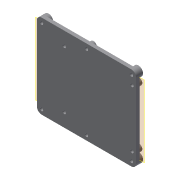
# Autodesk Inventor part: cellSTORM_v5_Electronicbox
Saved by Autodesk Inventor 2019 (Build 230136000, 136)
## iProperties
Created: 2020-05-04
Part Number: cellSTORM_v5_Electronicbox
Material: Generic
Document SubType Name: Modeling
Designer: diederichbenedict
Density: 1 g/cm^3
Appearance: Default
Author: diederichbenedict
Autodesk Inventor part; units mm, degrees
ref_plane "YZ Plane" through (0, 0, 0) normal (1, 0, 0) x (0, 1, 0)
ref_plane "XZ Plane" through (0, 0, 0) normal (0, 1, 0) x (-1, 0, 0)
ref_plane "XY Plane" through (0, 0, 0) normal (0, 0, 1) x (1, 0, 0)
ref_plane "Work Plane1" through (0, 0, 3.25) normal (0, 0, 1) x (1, 0, 0)
sketch "Sketch1" plane through (0, 0, 3.25) normal (0, 0, 1) x (1, 0, 0)
  arc A0 (3, 0) -> (0, -3) centre (3, -3) ccw construction
  arc A1 (81.9242, -56) -> (84.9242, -53) centre (81.9242, -53) ccw construction
  arc A2 (84.9242, -3) -> (81.9242, 0) centre (81.9242, -3) ccw construction
  arc A3 (0, -53) -> (3, -56) centre (3, -53) ccw construction
  line L0 (0, 0) -> (86.0371, 0) construction
  line L1 (86.0371, 0) -> (86.0371, -52.7339) construction
  line L2 (86.0371, -52.7339) -> (0, -52.7339) construction
  line L3 (0, -52.7339) -> (0, 0) construction
  line L4 (80.9242, -64) -> (4, -64)
  line L5 (0, -60) -> (0, 4)
  line L6 (4, 8) -> (80.9242, 8)
  line L7 (84.9242, 4) -> (84.9242, -60)
  circle A4 centre (23.4242, -3.5) radius 1.375 projected
  circle A5 centre (23.4242, -52.5) radius 1.375 projected
  circle A6 centre (81.4242, -52.5) radius 1.375 projected
  circle A7 centre (81.4242, -3.5) radius 1.375 projected
  arc A8 (4, 8) -> (0, 4) centre (4, 4) ccw
  arc A9 (0, -60) -> (4, -64) centre (4, -60) ccw
  arc A10 (80.9242, -64) -> (84.9242, -60) centre (80.9242, -60) ccw
  arc A11 (84.9242, 4) -> (80.9242, 8) centre (80.9242, 4) ccw
  circle A12 centre (42.4621, 4) radius 1.4
  circle A13 centre (4, 4) radius 1.4
  circle A14 centre (4, -60) radius 1.4
  circle A15 centre (42.4621, -60) radius 1.4
  circle A16 centre (80.9242, -60) radius 1.4
  circle A17 centre (80.9242, 4) radius 1.4
  point P0 (84.9242, -64)
  point P1 (0, 8)
  point P2 (0, -64)
  point P3 (84.9242, 8)
  dimension "d0" = 8
  dimension "d2" = 0
  dimension "d5" = 4
  dimension "d12" = 8
  dimension "d13" = 2.8
  dimension "d14" = 2.8
  dimension "d15" = 2.8
  dimension "d16" = 2.8
  dimension "d17" = 2.8
  dimension "d18" = 2.8
  constraints: 16 end point, 10 centre point, 8 point on circle, 8 point on line, 8 tangent, 6 coincident, 4 parallel, 3 equal radius, 2 horizontal, 2 perpendicular
  measures "d0" distance between parallel lines of L6 L0
  measures "d2" distance from line of A1.end L7
  measures "d5" radius of A8
  measures "d12" vertical distance of A3.end L4.end
  measures "d13" diameter of A12
  measures "d14" diameter of A13
  measures "d15" diameter of A14
  measures "d16" diameter of A15
  measures "d17" diameter of A16
  measures "d18" diameter of A17
extrude "Extrusion1" add sketch "Sketch1" along normal blind 3
sketch "Sketch2" plane through (0, 0, 3.25) normal (0, 0, -1) x (-1, 0, 0)
  circle A0 centre (-23.4242, -3.5) radius 1.375 projected
  circle A1 centre (-23.4242, -52.5) radius 1.375 projected
  arc A2 (-3, -56) -> (0, -53) centre (-3, -53) ccw projected
  line L0 (0, -3) -> (0, -53) projected
  arc A3 (0, -3) -> (-3, 0) centre (-3, -3) ccw projected
  line L1 (-81.9242, 0) -> (-3, 0) projected
  arc A4 (-81.9242, 0) -> (-84.9242, -3) centre (-81.9242, -3) ccw projected
  line L2 (-84.9242, -53) -> (-84.9242, -3) projected
  arc A5 (-84.9242, -53) -> (-81.9242, -56) centre (-81.9242, -53) ccw projected
  line L3 (-3, -56) -> (-81.9242, -56) projected
  circle A6 centre (-22.213, -8.2226) radius 0.5 projected
  circle A7 centre (-24.7543, -8.2226) radius 0.5 projected
  circle A8 centre (-67.0848, -6.0884) radius 0.2 projected
  circle A9 centre (-48.353, -16.7207) radius 0.2 projected
  circle A10 centre (-47.3865, -17.6798) radius 0.2 projected
  circle A11 centre (-45.8783, -17.6652) radius 0.2 projected
  circle A12 centre (-44.8533, -17.6652) radius 0.2 projected
  circle A13 centre (-46.2005, -16.2668) radius 0.2 projected
  circle A14 centre (-45.5781, -16.2009) radius 0.2 projected
  circle A15 centre (-44.9045, -16.1936) radius 0.2 projected
  circle A16 centre (-44.2822, -16.3107) radius 0.2 projected
  circle A17 centre (-43.9225, -35.8663) radius 0.2 projected
  circle A18 centre (-43.7816, -34.9329) radius 0.2 projected
  circle A19 centre (-44.7326, -34.6159) radius 0.2 projected
  circle A20 centre (-46.2119, -33.2071) radius 0.2 projected
  circle A21 centre (-43.4822, -31.4107) radius 0.2 projected
  circle A22 centre (-38.8402, -21.8362) radius 0.2 projected
  circle A23 centre (-38.8242, -20.7804) radius 0.2 projected
  circle A24 centre (-36.9127, -18.1491) radius 0.2 projected
  circle A25 centre (-37.5765, -17.9571) radius 0.2 projected
  circle A26 centre (-37.0167, -19.0928) radius 0.2 projected
  circle A27 centre (-38.1204, -19.9646) radius 0.2 projected
  line L4 (-38.4822, -15.9107) -> (-37.8289, -15.9107) projected
  line L5 (-37.8289, -16.3532) -> (-37.8289, -15.9107) projected
  line L6 (-37.8289, -16.3532) -> (-38.4822, -16.3532) projected
  line L7 (-38.4822, -15.9107) -> (-38.4822, -16.3532) projected
  line L8 (-38.5091, -16.758) -> (-37.8127, -16.758) projected
  line L9 (-37.8127, -17.341) -> (-37.8127, -16.758) projected
  line L10 (-37.8127, -17.341) -> (-38.5091, -17.341) projected
  line L11 (-38.5091, -16.758) -> (-38.5091, -17.341) projected
  circle A28 centre (-72.081, -8.9661) radius 0.2 projected
  circle A29 centre (-79.5495, -9.7485) radius 0.2 projected
  circle A30 centre (-79.9051, -8.7527) radius 0.2 projected
  circle A31 centre (-77.6646, -9.4996) radius 0.2 projected
  circle A32 centre (-79.7806, -11.3489) radius 0.2 projected
  circle A33 centre (-79.3894, -12.807) radius 0.2 projected
  circle A34 centre (-79.1761, -13.5361) radius 0.2 projected
  circle A35 centre (-70.8491, -11.3341) radius 0.2 projected
  circle A36 centre (-70.7681, -10.4839) radius 0.2 projected
  circle A37 centre (-71.8713, -11.4758) radius 0.2 projected
  circle A38 centre (-47.3628, -8.6438) radius 0.2 projected
  circle A39 centre (-67.9301, -8.3536) radius 0.2 projected
  circle A40 centre (-68.8541, -7.4295) radius 0.2 projected
  circle A41 centre (-64.6394, -6.3589) radius 0.2 projected
  circle A42 centre (-65.124, -8.6691) radius 0.2 projected
  circle A43 centre (-67.1863, -9.0861) radius 0.2 projected
  circle A44 centre (-66.6003, -9.8073) radius 0.2 projected
  circle A45 centre (-66.7693, -10.5962) radius 0.2 projected
  circle A46 centre (-66.8031, -11.2611) radius 0.2 projected
  circle A47 centre (-65.586, -10.9681) radius 0.2 projected
  circle A48 centre (-62.3629, -10.461) radius 0.2 projected
  circle A49 centre (-62.4756, -12.7825) radius 0.2 projected
  circle A50 centre (-64.7183, -13.8643) radius 0.2 projected
  circle A51 centre (-63.873, -13.8643) radius 0.2 projected
  circle A52 centre (-61.9347, -16.2197) radius 0.2 projected
  circle A53 centre (-59.9625, -15.3068) radius 0.2 projected
  circle A54 centre (-60.7965, -14.1573) radius 0.2 projected
  circle A55 centre (-58.7116, -11.0019) radius 0.2 projected
  circle A56 centre (-56.2098, -8.2183) radius 0.2 projected
  circle A57 centre (-55.1542, -11.3073) radius 0.2 projected
  circle A58 centre (-58.4406, -13.9483) radius 0.2 projected
  circle A59 centre (-57.6689, -13.9483) radius 0.2 projected
  circle A60 centre (-56.7841, -14.2211) radius 0.2 projected
  circle A61 centre (-56.345, -11.3738) radius 0.2 projected
  circle A62 centre (-43.0801, -22.1797) radius 0.2 projected
  circle A63 centre (-45.846, -22.8336) radius 0.2 projected
  circle A64 centre (-45.6957, -23.6153) radius 0.2 projected
  circle A65 centre (-47.4169, -23.2545) radius 0.2 projected
  circle A66 centre (-47.3794, -24.8404) radius 0.2 projected
  circle A67 centre (-47.7852, -23.7957) radius 0.2 projected
  circle A68 centre (-46.0339, -25.0509) radius 0.2 projected
  circle A69 centre (-37.8814, -28.3476) radius 0.2 projected
  circle A70 centre (-38.5166, -28.276) radius 0.2 projected
  circle A71 centre (-39.2056, -28.3208) radius 0.2 projected
  circle A72 centre (-38.123, -26.8266) radius 0.2 projected
  circle A73 centre (-38.9819, -26.8266) radius 0.2 projected
  circle A74 centre (-39.134, -25.3146) radius 0.2 projected
  circle A75 centre (-45.0926, -23.6057) radius 0.2 projected
  circle A76 centre (-39.805, -25.3146) radius 0.2 projected
  circle A77 centre (-40.306, -25.8693) radius 0.2 projected
  circle A78 centre (-73.2524, -44.2624) radius 0.2 projected
  circle A79 centre (-75.8766, -48.3708) radius 0.2 projected
  circle A80 centre (-74.335, -47.9589) radius 0.2 projected
  circle A81 centre (-75.6234, -44.5695) radius 0.2 projected
  circle A82 centre (-60.44, -36.6138) radius 0.2 projected
  circle A83 centre (-61.037, -35.3004) radius 0.2 projected
  circle A84 centre (-61.2076, -34.3622) radius 0.2 projected
  circle A85 centre (-64.6361, -37.0573) radius 0.2 projected
  circle A86 centre (-65.3014, -36.0338) radius 0.2 projected
  circle A87 centre (-64.6703, -33.3899) radius 0.2 projected
  circle A88 centre (-63.715, -39.9741) radius 0.2 projected
  circle A89 centre (-65.1479, -39.0018) radius 0.2 projected
  circle A90 centre (-68.8954, -35.575) radius 0.2 projected
  circle A91 centre (-69.402, -34.9183) radius 0.2 projected
  circle A92 centre (-69.8898, -36.0628) radius 0.2 projected
  circle A93 centre (-72.1039, -38.1643) radius 0.2 projected
  circle A94 centre (-71.935, -41.8794) radius 0.2 projected
  circle A95 centre (-72.1227, -34.7119) radius 0.2 projected
  circle A96 centre (-74.0553, -35.256) radius 0.2 projected
  circle A97 centre (-75.0685, -34.9558) radius 0.2 projected
  circle A98 centre (-77.5077, -35.1622) radius 0.2 projected
  circle A99 centre (-68.9517, -32.6104) radius 0.2 projected
  circle A100 centre (-66.6813, -30.8654) radius 0.2 projected
  circle A101 centre (-66.8877, -29.6458) radius 0.2 projected
  circle A102 centre (-44.52, -23.6415) radius 0.2 projected
  circle A103 centre (-45.0568, -24.8404) radius 0.2 projected
  circle A104 centre (-44.4842, -24.8225) radius 0.2 projected
  circle A105 centre (-43.8937, -24.8136) radius 0.2 projected
  circle A106 centre (-42.3638, -26.2988) radius 0.2 projected
  circle A107 centre (-43.7148, -26.2719) radius 0.2 projected
  circle A108 centre (-44.7079, -26.2719) radius 0.2 projected
  circle A109 centre (-44.1979, -26.7193) radius 0.2 projected
  circle A110 centre (-44.7705, -26.8445) radius 0.2 projected
  circle A111 centre (-41.5854, -28.2402) radius 0.2 projected
  circle A112 centre (-42.9543, -28.2134) radius 0.2 projected
  circle A113 centre (-44.2695, -28.3118) radius 0.2 projected
  circle A114 centre (-44.9763, -28.4192) radius 0.2 projected
  circle A115 centre (-45.3968, -26.6656) radius 0.2 projected
  circle A116 centre (-46.0142, -26.7551) radius 0.2 projected
  circle A117 centre (-47.6514, -26.3882) radius 0.2 projected
  circle A118 centre (-48.8593, -27.5961) radius 0.2 projected
  circle A119 centre (-55.7434, -31.6719) radius 0.2 projected
  circle A120 centre (-57.2346, -31.7216) radius 0.2 projected
  circle A121 centre (-56.4393, -32.9394) radius 0.2 projected
  circle A122 centre (-70.5072, -27.1836) radius 0.2 projected
  circle A123 centre (-82.0135, -8.0436) radius 0.2 projected
  circle A124 centre (-77.8638, -7.5634) radius 0.2 projected
  circle A125 centre (-77.3837, -6.7061) radius 0.2 projected
  circle A126 centre (-69.7875, -6.2774) radius 0.2 projected
  circle A127 centre (-70.8849, -6.6203) radius 0.2 projected
  circle A128 centre (-70.2762, -8.4294) radius 0.2 projected
  circle A129 centre (-72.6339, -6.5603) radius 0.2 projected
  circle A130 centre (-77.2174, -15.0208) radius 0.2 projected
  circle A131 centre (-74.5254, -13.0345) radius 0.2 projected
  circle A132 centre (-74.7215, -13.6095) radius 0.2 projected
  circle A133 centre (-74.2641, -14.1061) radius 0.2 projected
  circle A134 centre (-74.826, -14.6941) radius 0.2 projected
  circle A135 centre (-71.0103, -13.8709) radius 0.2 projected
  circle A136 centre (-70.9057, -14.6027) radius 0.2 projected
  circle A137 centre (-72.8789, -14.7856) radius 0.2 projected
  circle A138 centre (-72.2909, -15.1646) radius 0.2 projected
  circle A139 centre (-76.4202, -23.4755) radius 0.2 projected
  circle A140 centre (-76.6424, -22.9136) radius 0.2 projected
  circle A141 centre (-72.1341, -21.5546) radius 0.2 projected
  circle A142 centre (-71.337, -21.5938) radius 0.2 projected
  circle A143 centre (-75.414, -19.4507) radius 0.2 projected
  circle A144 centre (-77.335, -18.9933) radius 0.2 projected
  circle A145 centre (-73.0619, -16.7196) radius 0.2 projected
  circle A146 centre (-72.1733, -16.1838) radius 0.2 projected
  circle A147 centre (-70.7751, -16.1316) radius 0.2 projected
  circle A148 centre (-70.7881, -17.0724) radius 0.2 projected
  circle A149 centre (-71.7558, -44.5458) radius 0.2 projected
  circle A150 centre (-66.535, -44.9267) radius 0.2 projected
  circle A151 centre (-65.8404, -45.218) radius 0.2 projected
  circle A152 centre (-64.1151, -43.2014) radius 0.2 projected
  circle A153 centre (-67.1848, -42.3948) radius 0.2 projected
  circle A154 centre (-68.2379, -42.4172) radius 0.2 projected
  circle A155 centre (-80.9558, -44.2504) radius 0.2 projected
  circle A156 centre (-80.0692, -44.0164) radius 0.2 projected
  circle A157 centre (-83.899, -39.4107) radius 0.2 projected
  circle A158 centre (-83.9729, -38.6226) radius 0.2 projected
  circle A159 centre (-83.8374, -36.4183) radius 0.2 projected
  circle A160 centre (-78.5914, -39.5092) radius 0.2 projected
  circle A161 centre (-78.5791, -38.1177) radius 0.2 projected
  circle A162 centre (-77.8266, -25.7432) radius 0.2 projected
  circle A163 centre (-77.9087, -28.671) radius 0.2 projected
  circle A164 centre (-77.895, -31.7083) radius 0.2 projected
  circle A165 centre (-74.0916, -28.6573) radius 0.2 projected
  circle A166 centre (-77.6854, -23.1009) radius 0.2 projected
  circle A167 centre (-75.7973, -21.5412) radius 0.2 projected
  circle A168 centre (-70.7489, -18.0525) radius 0.2 projected
  circle A169 centre (-70.8584, -18.9144) radius 0.2 projected
  circle A170 centre (-70.7763, -19.5301) radius 0.2 projected
  circle A171 centre (-66.4667, -19.749) radius 0.2 projected
  circle A172 centre (-65.6666, -20.7133) radius 0.2 projected
  circle A173 centre (-71.5914, -22.7486) radius 0.2 projected
  circle A174 centre (-71.4444, -23.5627) radius 0.2 projected
  circle A175 centre (-72.2443, -23.8456) radius 0.2 projected
  circle A176 centre (-73.4429, -24.8971) radius 0.2 projected
  circle A177 centre (-68.4368, -27.26) radius 0.2 projected
  circle A178 centre (-73.2535, -29.6345) radius 0.2 projected
  circle A179 centre (-73.1065, -28.6847) radius 0.2 projected
  circle A180 centre (-71.125, -25.1459) radius 0.2 projected
  circle A181 centre (-71.1935, -25.8197) radius 0.2 projected
  circle A182 centre (-71.2849, -27.2245) radius 0.2 projected
  circle A183 centre (-71.1706, -29.5087) radius 0.2 projected
  circle A184 centre (-71.2278, -28.6864) radius 0.2 projected
  circle A185 centre (-66.8649, -27.1446) radius 0.2 projected
  circle A186 centre (-66.6593, -28.8235) radius 0.2 projected
  circle A187 centre (-66.5108, -30.2625) radius 0.2 projected
  circle A188 centre (-42.5801, -10.5439) radius 0.2 projected
  circle A189 centre (-41.6928, -10.461) radius 0.2 projected
  circle A190 centre (-40.7805, -10.4527) radius 0.2 projected
  circle A191 centre (-44.6203, -13.488) radius 0.2 projected
  circle A192 centre (-42.0825, -14.4002) radius 0.2 projected
  circle A193 centre (-45.491, -12.3933) radius 0.2 projected
  circle A194 centre (-44.5373, -12.4265) radius 0.2 projected
  circle A195 centre (-43.426, -12.4099) radius 0.2 projected
  circle A196 centre (-0.8218, -17.9959) radius 0.2 projected
  circle A197 centre (-5.3083, -17.8009) radius 0.2 projected
  circle A198 centre (-36.7643, -43.1201) radius 0.2 projected
  circle A199 centre (-19.8744, -38.9768) radius 0.2 projected
  circle A200 centre (-20.6732, -38.164) radius 0.2 projected
  circle A201 centre (-16.553, -31.5352) radius 0.2 projected
  circle A202 centre (-16.6371, -33.7074) radius 0.2 projected
  circle A203 centre (-17.4359, -35.4873) radius 0.2 projected
  circle A204 centre (-20.477, -31.0167) radius 0.2 projected
  circle A205 centre (-21.5701, -33.8896) radius 0.2 projected
  circle A206 centre (-31.4223, -28.9566) radius 0.2 projected
  circle A207 centre (-29.5724, -29.9936) radius 0.2 projected
  circle A208 centre (-28.8156, -27.3589) radius 0.2 projected
  circle A209 centre (-27.8906, -27.401) radius 0.2 projected
  circle A210 centre (-26.3911, -27.5551) radius 0.2 projected
  circle A211 centre (-24.8635, -27.485) radius 0.2 projected
  circle A212 centre (-24.1564, -30.0892) radius 0.2 projected
  circle A213 centre (-23.9144, -29.4776) radius 0.2 projected
  circle A214 centre (-22.8697, -30.1147) radius 0.2 projected
  circle A215 centre (-23.2009, -29.5541) radius 0.2 projected
  circle A216 centre (-23.1499, -27.4901) radius 0.2 projected
  circle A217 centre (-22.3218, -27.4901) radius 0.2 projected
  circle A218 centre (-21.2899, -27.401) radius 0.2 projected
  circle A219 centre (-20.5113, -27.5708) radius 0.2 projected
  circle A220 centre (-19.7893, -23.9044) radius 0.2 projected
  circle A221 centre (-19.761, -21.3705) radius 0.2 projected
  circle A222 centre (-19.4779, -20.7335) radius 0.2 projected
  circle A223 centre (-19.7893, -18.7941) radius 0.2 projected
  circle A224 centre (-19.945, -17.8598) radius 0.2 projected
  circle A225 centre (-21.2757, -16.7698) radius 0.2 projected
  circle A226 centre (-22.3799, -15.5949) radius 0.2 projected
  circle A227 centre (-24.7014, -15.6232) radius 0.2 projected
  circle A228 centre (-29.8825, -15.7648) radius 0.2 projected
  circle A229 centre (-35.6443, -10.4124) radius 0.2 projected
  circle A230 centre (-37.175, -12.1575) radius 0.2 projected
  circle A231 centre (-39.8268, -12.6255) radius 0.2 projected
  circle A232 centre (-37.331, -14.1464) radius 0.2 projected
  circle A233 centre (-37.0872, -14.8191) radius 0.2 projected
  circle A234 centre (-38.3839, -15.2773) radius 0.2 projected
  circle A235 centre (-38.9688, -15.9012) radius 0.2 projected
  circle A236 centre (-40.636, -16.2522) radius 0.2 projected
  circle A237 centre (-41.2794, -16.301) radius 0.2 projected
  circle A238 centre (-39.7721, -19.9788) radius 0.2 projected
  circle A239 centre (-41.478, -19.3199) radius 0.2 projected
  circle A240 centre (-42.2322, -19.9715) radius 0.2 projected
  circle A241 centre (-47.1376, -20.7183) radius 0.2 projected
  circle A242 centre (-44.8753, -21.326) radius 0.2 projected
  circle A243 centre (-45.7392, -20.8208) radius 0.2 projected
  circle A244 centre (-44.824, -20.7549) radius 0.2 projected
  circle A245 centre (-46.0467, -19.8031) radius 0.2 projected
  circle A246 centre (-45.439, -19.6201) radius 0.2 projected
  circle A247 centre (-44.4579, -19.686) radius 0.2 projected
  circle A248 centre (-44.7654, -19.1442) radius 0.2 projected
  circle A249 centre (-44.0479, -19.0417) radius 0.2 projected
  circle A250 centre (-42.364, -18.024) radius 0.2 projected
  circle A251 centre (-44.6117, -18.5511) radius 0.2 projected
  circle A252 centre (-47.3353, -19.254) radius 0.2 projected
  circle A253 centre (-42.3786, -18.844) radius 0.2 projected
  circle A254 centre (-45.8856, -18.4999) radius 0.2 projected
  circle A255 centre (-73.3884, -7.7263) radius 0.2 projected
  circle A256 centre (-73.2512, -8.8838) radius 0.2 projected
  circle A257 centre (-72.7822, -10.7673) radius 0.2 projected
  circle A258 centre (-72.747, -11.7788) radius 0.2 projected
  circle A259 centre (-73.7231, -11.767) radius 0.2 projected
  circle A260 centre (-76.5692, -10.5556) radius 0.2 projected
  circle A261 centre (-76.5339, -11.1437) radius 0.2 projected
  circle A262 centre (-76.7103, -12.1669) radius 0.2 projected
  circle A263 centre (-78.9449, -14.3897) radius 0.2 projected
  circle A264 centre (-72.9965, -18.0002) radius 0.2 projected
  circle A265 centre (-73.271, -19.5945) radius 0.2 projected
  circle A266 centre (-78.1452, -14.1192) radius 0.2 projected
  circle A267 centre (-77.4395, -14.1061) radius 0.2 projected
  circle A268 centre (-78.4065, -15.831) radius 0.2 projected
  circle A269 centre (-78.3673, -16.6412) radius 0.2 projected
  circle A270 centre (-77.8969, -17.4514) radius 0.2 projected
  circle A271 centre (-77.2304, -16.7065) radius 0.2 projected
  circle A272 centre (-76.2112, -15.5174) radius 0.2 projected
  circle A273 centre (-76.5901, -16.4321) radius 0.2 projected
  circle A274 centre (-77.0605, -15.7918) radius 0.2 projected
  circle A275 centre (-55.7793, -42.2185) radius 0.2 projected
  circle A276 centre (-57.5522, -41.3263) radius 0.2 projected
  circle A277 centre (-55.928, -40.3426) radius 0.2 projected
  circle A278 centre (-55.8365, -41.4178) radius 0.2 projected
  circle A279 centre (-55.8822, -43.1107) radius 0.2 projected
  circle A280 centre (-58.7419, -42.127) radius 0.2 projected
  circle A281 centre (-59.3824, -38.5924) radius 0.2 projected
  circle A282 centre (-65.8036, -48.151) radius 0.2 projected
  circle A283 centre (-62.4709, -42.9163) radius 0.2 projected
  circle A284 centre (-62.8822, -51.3107) radius 0.2 projected
  circle A285 centre (-61.8658, -53.7387) radius 0.2 projected
  circle A286 centre (-61.9694, -54.7362) radius 0.2 projected
  circle A287 centre (-64.2185, -54.7268) radius 0.2 projected
  circle A288 centre (-66.016, -54.7927) radius 0.2 projected
  circle A289 centre (-64.3597, -51.1319) radius 0.2 projected
  circle A290 centre (-67.8605, -51.9789) radius 0.2 projected
  circle A291 centre (-64.7644, -49.7768) radius 0.2 projected
  circle A292 centre (-68.698, -51.8189) radius 0.2 projected
  circle A293 centre (-75.1352, -48.7709) radius 0.2 projected
  circle A294 centre (-81.4242, -3.5) radius 1.375 projected
  circle A295 centre (-81.4242, -52.5) radius 1.375 projected
  circle A296 centre (-23.4242, -52.5) radius 1.375 projected
  circle A297 centre (-23.4242, -3.5) radius 1.375 projected
  circle A298 centre (-75.669, -6.1316) radius 0.2 projected
  circle A299 centre (-81.4242, -3.5) radius 2.875
  circle A300 centre (-81.4242, -52.5) radius 2.875
  circle A301 centre (-23.4242, -52.5) radius 2.875
  circle A302 centre (-23.4242, -3.5) radius 2.875
  circle A303 centre (-4, 4) radius 1.4 projected
  circle A304 centre (-42.4621, 4) radius 1.4 projected
  circle A305 centre (-80.9242, 4) radius 1.4 projected
  circle A306 centre (-80.9242, -60) radius 1.4 projected
  circle A307 centre (-42.4621, -60) radius 1.4 projected
  circle A308 centre (-4, -60) radius 1.4 projected
  circle A309 centre (-4, 4) radius 4
  circle A310 centre (-42.4621, 4) radius 2.9
  circle A311 centre (-80.9242, 4) radius 4
  circle A312 centre (-4, -60) radius 4
  circle A313 centre (-42.4621, -60) radius 2.9
  circle A314 centre (-80.9242, -60) radius 4
  point P0 (0, 0)
  point P1 (-84.9242, -60)
  point P2 (-80.9242, 8)
  point P3 (-4, 8)
  point P4 (0, -60)
  dimension "d6" = 1.5
  dimension "d7" = 1.5
  dimension "d8" = 1.5
  dimension "d9" = 1.5
  dimension "d20" = 1.5
  dimension "d23" = 1.5
  constraints: 6 centre point, 2 horizontal alignment, 2 vertical alignment, 8 other
  measures "d6" radial gap between concentric circles of A294 A299
  measures "d7" radial gap between concentric circles of A295 A300
  measures "d8" radial gap between concentric circles of A1 A301
  measures "d9" radial gap between concentric circles of A0 A302
  measures "d20" radial gap between concentric circles of A304 A310
  measures "d23" radial gap between concentric circles of A307 A313
extrude "Extrusion2" add sketch "Sketch2" along normal blind 3 contours A312 | A314 | A311 | A309 | A299 | A300 | A301 | A302 | A310 | A313
body "Solid1"
